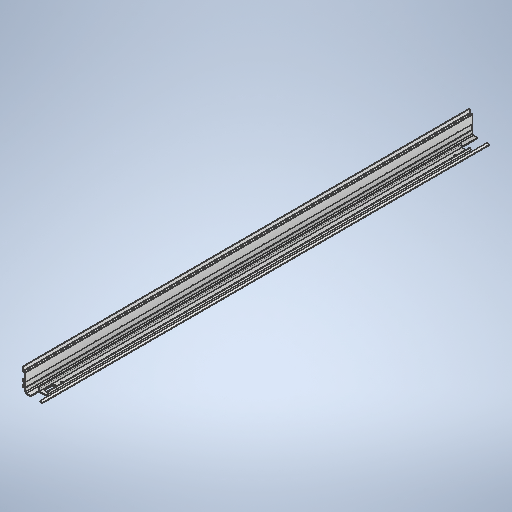
# Autodesk Inventor part: SP40-11 TAPETA - ENCUENTRO HOJA CORREDERA 695 mm
Saved by Autodesk Inventor 2025 (Build 290162000, 162)
## iProperties
Created: 2026-01-28
Part Number: SP40-11 TAPETA - ENCUENTRO HOJA CORREDERA 695 mm
Material: Aluminio
Document SubType Name: Modeling
Designer: ROLANDO
Density: 2.7 g/cm^3
Appearance: Satinado
Author: ROLANDO
Autodesk Inventor part; units mm, degrees
ref_plane "YZ Plane" through (0, 0, 0) normal (1, 0, 0) x (0, 1, 0)
ref_plane "XZ Plane" through (0, 0, 0) normal (0, 1, 0) x (-1, 0, 0)
ref_plane "XY Plane" through (0, 0, 0) normal (0, 0, 1) x (1, 0, 0)
sketch "Boceto1" plane through (0, 0, 0) normal (0, 0, 1) x (1, 0, 0)
  line L0 (2.8, 0) -> (27.3, 0)
  line L1 (27.8, 0.5) -> (27.8, 1.3)
  line L2 (0.5, 7.7) -> (1.3, 7.7)
  line L3 (0.5, 7.7) -> (0.5, 15.7)
  line L4 (0.5, 15.7) -> (1.3, 15.7)
  line L5 (1.3, 15.7) -> (1.3, 28.3)
  line L6 (0, 6.4) -> (-3.7, 6.4)
  line L7 (-3.7, 6.4) -> (-3.7, 9.7)
  line L8 (-3.7, 9.7) -> (-2.4, 9.7)
  line L9 (-2.4, 9.7) -> (-2.4, 7.7)
  line L10 (-2.4, 7.7) -> (-1.1, 7.7)
  line L11 (-1.1, 7.7) -> (-1.1, 15.7)
  line L12 (-1.1, 15.7) -> (-2.4, 15.7)
  line L13 (-2.4, 15.7) -> (-2.4, 13.7)
  line L14 (-2.4, 13.7) -> (-3.7, 13.7)
  line L15 (-3.7, 13.7) -> (-3.7, 17)
  line L16 (-3.7, 17) -> (0, 17)
  line L17 (0, 17) -> (0, 27)
  line L18 (0, 6.4) -> (0, 2.8)
  line L19 (0.8, 28.8) -> (-1.7379, 28.8)
  line L20 (-2.2319, 29.2226) -> (-2.98, 34)
  line L21 (-2.98, 34) -> (-3.7, 34)
  line L22 (-3.7, 34) -> (-3.7, 28)
  line L23 (-3.2, 27.5) -> (-0.5, 27.5)
  line L24 (1.3, 7.7) -> (1.3, 2.8)
  line L25 (9.1, 1.3) -> (9.1, 4.7)
  line L26 (10.1, 7.4376) -> (10.1, 1.3)
  line L27 (22.5, 1.3) -> (22.5, 7.4376)
  line L28 (23.5, 4.7) -> (23.5, 1.3)
  line L29 (23.5, 1.3) -> (27.8, 1.3)
  line L30 (2.8, 1.3) -> (9.1, 1.3)
  line L31 (10.1, 1.3) -> (22.5, 1.3)
  arc A0 (0, 2.8) -> (2.8, 0) centre (2.8, 2.8) ccw
  arc A1 (27.3, 0) -> (27.8, 0.5) centre (27.3, 0.5) ccw
  arc A2 (0, 27) -> (-0.5, 27.5) centre (-0.5, 27) ccw
  arc A3 (-3.7, 28) -> (-3.2, 27.5) centre (-3.2, 28) ccw
  arc A4 (1.3, 28.3) -> (0.8, 28.8) centre (0.8, 28.3) ccw
  arc A5 (-2.2319, 29.2226) -> (-1.7379, 28.8) centre (-1.7379, 29.3) ccw
  arc A6 (1.3, 2.8) -> (2.8, 1.3) centre (2.8, 2.8) ccw
  line L32 (23.5, 4.7) -> (24.4, 4.9649)
  line L33 (24.4, 4.9649) -> (23.5, 7.4376)
  line L34 (9.1, 4.7) -> (8.2, 4.9649)
  line L35 (8.2, 4.9649) -> (9.1, 7.4376)
  line L36 (23.5, 10.0894) -> (23.5, -1.1197) construction
  line L37 (23.5, 7.4376) -> (22.5, 7.4376)
  line L38 (9.1, 10.0894) -> (9.1, -1.1197) construction
  line L39 (9.1, 7.4376) -> (10.1, 7.4376)
  point P0 (0, 0)
  point P1 (-1.1, 11.7)
  dimension "d3" = 1.3
  dimension "d4" = 1.3
  dimension "d6" = 1.3
  dimension "d7" = 1.3
  dimension "d9" = 1.3
  dimension "d10" = 1.3
  dimension "d11" = 1.3
  dimension "d15" = 34
  dimension "d16" = 31.5
  dimension "d44" = 6.4
  dimension "d45" = 4
  dimension "d46" = 8
  dimension "d47" = 2
  dimension "d48" = 10.6
  dimension "d49" = 1.3
  dimension "d51" = 0.8
  dimension "d52" = 0.8
  dimension "d53" = 6.5
  dimension "d57" = 98.9
  dimension "d58" = 0.72
  dimension "d60" = 1.6
  dimension "d61" = 2.8
  dimension "d63" = 0.5
  dimension "d64" = 0.5
  dimension "d65" = 31.5
  dimension "d70" = 1.5
  dimension "d71" = 1.3
  dimension "d77" = 3.4
  dimension "d78" = 3.4
  dimension "d80" = 4.3
  dimension "d83" = 16.4
  dimension "d86" = 0.9
  dimension "d87" = 16.4
  dimension "d92" = 70
  dimension "d94" = 1
  dimension "d95" = 0.9
  dimension "d96" = 1
  dimension "d97" = 70
  dimension "d98" = 14.4
  dimension "d99" = 7.8
  dimension "d108" = 2.9
  constraints: 80 end point, 26 perpendicular, 14 point on circle, 14 tangent, 10 point on line, 7 centre point, 6 collinear, 6 horizontal, 5 vertical, 3 equal radius, 2 parallel, 1 midpoint
  measures "d3" distance between parallel lines of L0 L31
  measures "d4" distance between parallel lines of L18 L24
  measures "d6" distance between parallel lines of L10 L6
  measures "d7" distance between parallel lines of L7 L9
  measures "d9" distance between parallel lines of L16 L12
  measures "d10" distance between parallel lines of L17 L5
  measures "d11" distance between parallel lines of L19 L23
  measures "d15" distance between parallel lines of L21 L0
  measures "d16" distance between parallel lines of L7 L1
  measures "d44" distance between parallel lines of L0 L6
  measures "d45" distance between parallel lines of L14 L8
  measures "d46" distance between parallel lines of L10 L12
  measures "d47" distance from line of L14 point (-1.1, 11.7)
  measures "d48" distance between parallel lines of L6 L16
  measures "d49" distance between parallel lines of L11 L13
  measures "d51" distance of L2.start L2.end
  measures "d52" distance of L3.end L4.end
  measures "d53" distance between parallel lines of L23 L21
  measures "d57" angle of L19 L20
  measures "d58" distance of L20.end L21.end
  measures "d60" distance between parallel lines of L11 L3
  measures "d61" radius of A0
  measures "d63" radius of A1
  measures "d64" radius of A2
  measures "d65" distance between parallel lines of L1 L22
  measures "d70" radius of A6
  measures "d71" radial gap between concentric circles of A0 A6
  measures "d77" distance of L25.start L25.end
  measures "d78" distance of L28.start L28.end
  measures "d80" distance between parallel lines of L28 L1
  measures "d83" angle of L29 L32
  measures "d86" distance from line of L25 L34.end
  measures "d87" angle of L30 L34
  measures "d92" angle of L31 L33
  measures "d94" distance of L33.end L27.end
  measures "d95" distance from line of L36 L32.end
  measures "d96" distance between parallel lines of L26 L25
  measures "d97" angle of L31 L35
  measures "d98" distance between parallel lines of L28 L25
  measures "d99" distance between parallel lines of L24 L25
  measures "d108" horizontal distance of L32.end L0.end
extrude "Extrusión1" add sketch "Boceto1" against normal blind 695
sketch "Boceto4" plane through (2.8, 0, 0) normal (0, -1, 0) x (1, 0, 0)
  line L0 (0, 0) -> (24.5, 0) projected
  line L1 (20.7, 0) -> (6.3, 0)
  line L2 (6.3, 0) -> (6.3, -12.8)
  line L3 (6.3, -12.8) -> (20.7, -12.8)
  line L4 (20.7, -12.8) -> (20.7, 0)
  line L5 (24.5, 0) -> (24.5, -695) projected
  line L6 (0, 0) -> (0, -695) projected
  line L7 (13.5, -22.1) -> (13.5, -29.1) construction
  line L8 (18.5, -22.1) -> (18.5, -29.1)
  line L9 (8.5, -29.1) -> (8.5, -22.1)
  arc A0 (18.5, -22.1) -> (8.5, -22.1) centre (13.5, -22.1) ccw
  arc A1 (8.5, -29.1) -> (18.5, -29.1) centre (13.5, -29.1) ccw
  circle A2 centre (13.5, -42.1) radius 2
  line L10 (13.5, -9.0915) -> (13.5, -53.7508) construction
  line L11 (25, 0) -> (25, -695) projected
  line L12 (20.7, -695) -> (6.3, -695)
  line L13 (6.3, -695) -> (6.3, -669.4)
  line L14 (6.3, -669.4) -> (20.7, -669.4)
  line L15 (20.7, -669.4) -> (20.7, -695)
  line L16 (24.5, -695) -> (0, -695) projected
  circle A3 centre (13.5, -652.9) radius 2
  point P0 (-2.8, 0)
  point P1 (13.5, -25.6)
  point P2 (13.5, -34.1)
  point P3 (13.5, -17.1)
  point P4 (13.5, -12.8)
  dimension "d109" = 12.8
  dimension "d114" = 10
  dimension "d115" = 17
  dimension "d118" = 4.3
  dimension "d121" = 4
  dimension "d125" = 14.4
  dimension "d126" = 4.3
  dimension "d127" = 8
  dimension "d131" = 4.3
  dimension "d132" = 14.4
  dimension "d133" = 25.6
  dimension "d134" = 4
  dimension "d135" = 16.5
  dimension "d136" = 11.5
  constraints: 26 end point, 6 point on circle, 5 parallel, 5 point on line, 4 centre point, 4 tangent, 2 horizontal, 2 midpoint, 2 perpendicular, 2 vertical
  measures "d109" distance of L3.end L1.start
  measures "d114" distance between parallel lines of L9 L8
  measures "d115" distance of point (13.5, -34.1) point (13.5, -17.1)
  measures "d118" distance from line of L3 point (13.5, -17.1)
  measures "d121" diameter of A2
  measures "d125" distance of L2.end L3.end
  measures "d126" distance between parallel lines of L4 L11
  measures "d127" distance of point (13.5, -34.1) A2.centre
  measures "d131" distance between parallel lines of L11 L15
  measures "d132" distance of L13.end L14.end
  measures "d133" distance of L12.end L13.end
  measures "d134" diameter of A3
  measures "d135" distance from line of L14 A3.centre
  measures "d136" distance from line of L11 A3.centre
extrude "Extrusión4" cut sketch "Boceto4" against normal through all contours L0 L4 L3 L2 | L13 L14 L15 L12 | L8 A1 L9 A0 | A2 | A3
ref_plane "Plano de trabajo3" through (0, 0, 0) normal (0, 0, 1) x (1, 0, 0)
sketch "Boceto5" plane through (0, 0, 0) normal (0, 0, 1) x (1, 0, 0)
  line L0 (24.4, 1.8205) -> (8.0624, 1.8205)
  line L1 (8.0624, 1.8205) -> (8.0624, 8.2042)
  line L2 (8.0624, 8.2042) -> (24.4, 8.2042)
  line L3 (24.4, 8.2042) -> (24.4, 1.8205)
  point P0 (0, 0)
  constraints: 8 end point, 2 parallel, 1 horizontal, 1 perpendicular
extrude "Extrusión5" cut sketch "Boceto5" against normal up to surface (12.8 mm away)
ref_plane "Plano de trabajo4" through (0, 0, -695) normal (0, 0, -1) x (-1, 0, 0)
sketch "Boceto6" plane through (0, 0, -695) normal (0, 0, -1) x (-1, 0, 0)
  line L0 (-9.1, 1.3) -> (-2.8, 1.3) projected
  line L1 (-7.3903, 1.3) -> (-24.6588, 1.3)
  line L2 (-24.6588, 1.3) -> (-24.6588, 8.0245)
  line L3 (-24.6588, 8.0245) -> (-7.3903, 8.0245)
  line L4 (-7.3903, 8.0245) -> (-7.3903, 1.3)
  point P0 (0, 0)
  constraints: 8 end point, 2 parallel, 1 horizontal, 1 perpendicular, 1 point on line
extrude "Extrusión6" cut sketch "Boceto6" against normal up to surface (25.6 mm away)
